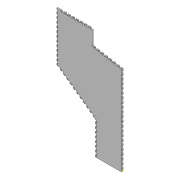
# Autodesk Inventor part: 00_Baseplate_Simmo_base
Saved by Autodesk Inventor 2022 (Build 260153000, 153)
## iProperties
Created: 2022-04-28
Part Number: 00_Baseplate_Simmo_base
Material: Generisch
Document SubType Name: Modeling
Designer: diederichbenedict
Density: 1 g/cm^3
Appearance: Vorgabe
Author: diederichbenedict
Autodesk Inventor part; units mm, degrees
ref_plane "YZ Plane" through (0, 0, 0) normal (1, 0, 0) x (0, 1, 0)
ref_plane "XZ Plane" through (0, 0, 0) normal (0, 1, 0) x (-1, 0, 0)
ref_plane "XY Plane" through (0, 0, 0) normal (0, 0, 1) x (1, 0, 0)
ref_plane "Arbeitsebene1" through (0, 0, 0) normal (0, 0, 1) x (1, 0, 0)
sketch "Skizze1" plane through (0, 0, 0) normal (0, 0, 1) x (1, 0, 0)
  line L0 (91.8818, 443.0401) -> (90.2278, 433.6598) projected
  line L1 (120, 0) -> (126, 0)
  line L2 (126, 0) -> (126, 440)
  line L3 (126, 440) -> (-21.6976, 466.0431)
  line L4 (-21.6976, 538.0431) -> (-196, 538.0431)
  line L5 (-196, 538.0431) -> (-196, 298.0431)
  line L6 (-196, 298.0431) -> (-6, 160)
  line L7 (-6, 160) -> (-6, 0)
  circle A0 centre (58.4, 5) radius 2.95 projected
  line L8 (120, 0) -> (0, 0) projected
  line L9 (0, 0) -> (0, 10) projected
  line L10 (120, 10) -> (0, 10) projected
  line L11 (120, 0) -> (120, 10) projected
  line L12 (120, 0) -> (0, 0)
  line L13 (126, 0) -> (-6, 0)
  line L14 (64.2504, 447.9123) -> (88.7659, 443.5895) construction
  line L15 (-112.6783, 286.0908) -> (-134.5219, 301.9611) construction
  line L16 (-134.4827, 366.1267) -> (-158.3225, 378.8026) construction
  line L17 (-21.6976, 466.0431) -> (-21.6976, 538.0431)
  point P0 (126, 5)
  dimension "d1" = 90
  dimension "d66" = 160
  dimension "d67" = 6
  dimension "d68" = 6
  dimension "d69" = 440
  dimension "d70" = 190
  dimension "d71" = 240
  dimension "d72" = 72
  constraints: 20 end point, 3 horizontal, 3 parallel, 1 perpendicular, 1 point on line, 1 vertical
  measures "d1" angle of L5 L4
  measures "d66" vertical distance of L1.start L6.end
  measures "d67" distance between parallel lines of L11 L2
  measures "d68" distance between parallel lines of L7 L9
  measures "d69" distance of L1.end L2.end
  measures "d70" distance between parallel lines of L5 L7
  measures "d71" distance of L4.end L5.end
  measures "d72" distance of L3.end L4.start
extrude "Extrusion1" add sketch "Skizze1" along normal blind 5 contours L11 L10 L9 L13 L7 L6 L5 L4 L17 L3 L2 L1 | L8 L9 L10 L11 | A0
sketch "Skizze2" plane through (0, 0, 0) normal (0, 0, -1) x (-1, 0, 0)
  line L0 (-126, 0) -> (-120, 0)
  line L1 (-120, 0) -> (-120, 10)
  line L2 (-120, 10) -> (-126, 10)
  line L3 (-126, 10) -> (-126, 0)
  circle A0 centre (-123, 15) radius 1.5
  point P0 (0, 0)
  dimension "d8" = 6
  dimension "d9" = 10
  dimension "d15" = 3
  dimension "d16" = 5
  constraints: 8 end point, 2 parallel, 2 point on line, 1 centre point, 1 horizontal, 1 perpendicular
  measures "d8" distance of L2.end L1.end
  measures "d9" distance of L1.end L0.end
  measures "d15" diameter of A0
  measures "d16" distance from line of A0.centre L2
extrude "Extrusion2" cut sketch "Skizze2" against normal through all
sketch "Skizze3" plane through (0, 0, 0) normal (0, 0, -1) x (-1, 0, 0)
  line L0 (196, 298.0431) -> (6, 160) projected
  line L1 (196, 538.0431) -> (196, 298.0431) projected
  line L2 (21.6976, 538.0431) -> (196, 538.0431) projected
  line L3 (-126, 440) -> (21.6976, 466.0431) projected
pattern_linear "Rechteckige Anordnung1" count 24 spacing 20 along (0, 1, 0) of "Extrusion2"
sketch "Skizze4" plane through (0, 0, 0) normal (0, 0, -1) x (-1, 0, 0)
  line L0 (-120, 441.058) -> (-110.1519, 442.7944)
  line L1 (-110.1519, 442.7944) -> (-109.11, 436.8856)
  line L2 (-109.11, 436.8856) -> (-118.9581, 435.1491)
  line L3 (-118.9581, 435.1491) -> (-120, 441.058)
  circle A0 centre (-104.7069, 440.7083) radius 1.5
  line L4 (-126, 440) -> (21.6976, 466.0431) projected
  line L5 (-120, 0) -> (-120, 9.8) projected
  point P0 (0, 0)
  dimension "d17" = 10
  dimension "d18" = 6
  dimension "d19" = 3
  dimension "d20" = 5
  dimension "d73" = 3
  constraints: 8 end point, 2 parallel, 2 point on line, 1 centre point, 1 collinear, 1 perpendicular
  measures "d17" distance of L1.end L2.end
  measures "d18" distance of L0.end L1.end
  measures "d19" diameter of A0
  measures "d20" distance from line of A0.centre L1
  measures "d73" distance from line of L2 A0.centre
extrude "Extrusion3" cut sketch "Skizze4" against normal through all
pattern_linear "Rechteckige Anordnung2" count 7 spacing 20 along (-0.9848078, 0.1736482, 0) of "Extrusion3"
sketch "Skizze5" plane through (0, 0, 0) normal (0, 0, -1) x (-1, 0, 0)
  line L0 (21.6976, 538.0431) -> (21.6976, 532.0431)
  line L1 (21.6976, 532.0431) -> (31.6976, 532.0431)
  line L2 (31.6976, 532.0431) -> (31.6976, 538.0431)
  line L3 (31.6976, 538.0431) -> (21.6976, 538.0431)
  circle A0 centre (36.6976, 535.0431) radius 1.5
  line L4 (21.6976, 538.0431) -> (196, 538.0431) projected
  point P0 (0, 0)
  dimension "d29" = 6
  dimension "d30" = 10
  dimension "d31" = 3
  dimension "d32" = 5
  constraints: 8 end point, 2 parallel, 1 centre point, 1 coincident, 1 collinear, 1 perpendicular
  measures "d29" distance of L0.start L0.end
  measures "d30" distance of L1.end L0.end
  measures "d31" diameter of A0
  measures "d32" distance from line of A0.centre L2
extrude "Extrusion4" cut sketch "Skizze5" against normal through all
pattern_linear "Rechteckige Anordnung3" count 8 spacing 20 along (-1, 0, 0) of "Extrusion4"
sketch "Skizze6" plane through (0, 0, 0) normal (0, 0, -1) x (-1, 0, 0)
  line L0 (196, 538.0431) -> (196, 298.0431) projected
  line L1 (196, 532.0431) -> (190, 532.0431)
  line L2 (190, 532.0431) -> (190, 522.0431)
  line L3 (190, 522.0431) -> (196, 522.0431)
  line L4 (196, 522.0431) -> (196, 532.0431)
  circle A0 centre (193, 517.0431) radius 1.5
  line L5 (31.6976, 538.0431) -> (196, 538.0431) projected
  point P0 (0, 0)
  point P1 (196, 344.793)
  point P2 (196, 522.0431)
  point P3 (191.6976, 538.0431)
  dimension "d31" = 3
  dimension "d38" = 6
  dimension "d39" = 10
  dimension "d40" = 3
  dimension "d41" = 5
  dimension "d74" = 6
  dimension "d75" = 3
  constraints: 6 end point, 2 horizontal, 1 centre point, 1 parallel, 1 point on line, 1 vertical, 3 other
  measures "d38" distance of L1.start L1.end
  measures "d39" distance of L3.start L1.end
  measures "d40" diameter of A0
  measures "d41" distance from line of A0.centre L3
  measures "d74" distance between parallel lines of L1 L5
  measures "d75" distance from line of A0.centre L4
extrude "Extrusion5" cut sketch "Skizze6" against normal through all
pattern_linear "Rechteckige Anordnung4" count 24 spacing 20 along (0, -1, 0) of "Extrusion5"
sketch "Skizze7" plane through (0, 0, 0) normal (0, 0, -1) x (-1, 0, 0)
  line L0 (196, 298.0431) -> (6, 160) projected
  line L1 (196, 298.0431) -> (6, 160) projected
  line L2 (189.121, 293.0452) -> (185.5942, 297.8993)
  line L3 (185.5942, 297.8993) -> (177.5041, 292.0214)
  line L4 (177.5041, 292.0214) -> (181.0308, 287.1673)
  line L5 (181.0308, 287.1673) -> (189.121, 293.0452)
  line L6 (189.121, 293.0452) -> (195.121, 293.0452) construction
  circle A0 centre (175.2223, 286.6554) radius 1.5
  point P0 (0, 0)
  point P1 (181.0308, 287.1673)
  point P2 (192.6247, 295.5908)
  point P3 (185.0759, 290.1062)
  point P4 (190, 302.0431)
  dimension "d47" = 6
  dimension "d49" = 10
  dimension "d50" = 3
  dimension "d51" = 5
  dimension "d76" = 3
  dimension "d77" = 6
  constraints: 10 end point, 2 parallel, 2 perpendicular, 1 centre point, 1 equal length, 1 horizontal, 1 midpoint, 1 point on line
  measures "d47" distance of L2.start L2.end
  measures "d49" distance of L3.end L2.end
  measures "d50" diameter of A0
  measures "d51" distance from line of L4 A0.centre
  measures "d76" distance from line of A0.centre L5
  measures "d77" distance from line of point (190, 302.043) L2
extrude "Extrusion6" cut sketch "Skizze7" against normal through all
pattern_linear "Rechteckige Anordnung5" count 11 spacing 20 along (0.809017, -0.5877853, 0) of "Extrusion6"
sketch "Skizze8" plane through (0, 0, 0) normal (0, 0, -1) x (-1, 0, 0)
  line L0 (0, 160) -> (0, 150)
  line L1 (0, 150) -> (4.7841, 150)
  circle A0 centre (3, 145) radius 1.5
  line L2 (6, 160) -> (6, 0) projected
  line L3 (0, 150) -> (6, 150)
  line L4 (6, 150) -> (6, 160)
  line L5 (6, 160) -> (0, 160)
  line L6 (0, 160) -> (0, 150)
  point P0 (0, 183.2478)
  point P1 (6, 150)
  dimension "d58" = 10
  dimension "d59" = 3
  dimension "d60" = 5
  constraints: 12 end point, 2 parallel, 1 centre point, 1 horizontal, 1 perpendicular
  measures "d58" distance of L0.end L0.start
  measures "d59" diameter of A0
  measures "d60" distance from line of A0.centre L1
extrude "Extrusion7" cut sketch "Skizze8" against normal through all
pattern_linear "Rechteckige Anordnung6" count 24 spacing 20 along (0, -1, 0) of "Extrusion7"
equation "\"d16\" = 0.5 * d9"
equation "\"d17\" = d9"
equation "\"d20\" = 0.5 * d9"
equation "\"d73\" = 0.5 * d18"
equation "\"d25\" = 2 * d9"
equation "\"d30\" = d9"
equation "\"d32\" = 0.5 * d9"
equation "\"d37\" = 2 * d9"
equation "\"d39\" = d9"
equation "\"d41\" = 0.5 * d9"
equation "\"d74\" = d18"
equation "\"d49\" = d9"
equation "\"d51\" = 0.5 * d9"
equation "\"d77\" = d18"
equation "\"d56\" = 2 * d9"
equation "\"d60\" = 0.5 * d9"
equation "\"d14\" = 2 * d9"
equation "\"d46\" = 2 * d9"
equation "\"d65\" = 2 * d9"
